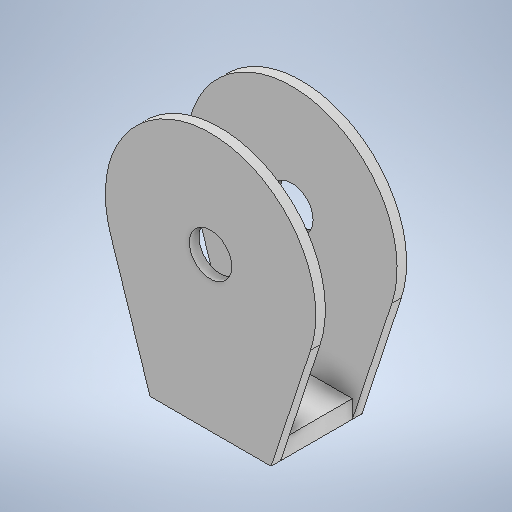
# Autodesk Inventor part: pulley
Saved by Autodesk Inventor 2025.2 (Build 292293000, 293)
## iProperties
Created: 2024-11-20
Part Number: pulley
Material: Generic
Document SubType Name: Modeling
Designer: email
Density: 1 g/cm^3
Appearance: Default
Author: email
Autodesk Inventor part; units mm, degrees
ref_plane "YZ Plane" through (0, 0, 0) normal (1, 0, 0) x (0, 1, 0)
ref_plane "XZ Plane" through (0, 0, 0) normal (0, 1, 0) x (-1, 0, 0)
ref_plane "XY Plane" through (0, 0, 0) normal (0, 0, 1) x (1, 0, 0)
sketch "Sketch1" plane through (0, 0, 0) normal (0, 0, 1) x (1, 0, 0)
  line L0 (0, 0) -> (25.3, 0)
  line L1 (25.3, 0) -> (25.3, 16.2986) construction
  line L2 (25.3, 16.2986) -> (0, 16.2986) construction
  line L3 (0, 16.2986) -> (0, 0) construction
  circle A0 centre (12.65, 32) radius 4.45
  circle A1 centre (12.65, 32) radius 22
  line L4 (25.3, 0) -> (33.5525, 25.138)
  line L5 (0, 0) -> (-8.2525, 25.138)
  line L6 (12.65, 54) -> (12.65, 0)
  dimension "d0" = 25.3
  dimension "d1" = 8.9
  dimension "d2" = 32
  dimension "d3" = 44
  dimension "d16" = 12.65
  constraints: 14 end point, 3 point on circle, 2 centre point, 2 parallel, 2 perpendicular, 2 tangent, 1 coincident, 1 horizontal, 1 midpoint, 1 point on line
  measures "d0" distance between parallel lines of L1 L3
  measures "d1" diameter of A0
  measures "d2" distance from line of L0 A0.centre
  measures "d3" diameter of A1
  measures "d16" distance between parallel lines of L1 L6
extrude "Extrusion1" add sketch "Sketch1" along normal blind 2 contours L5 A1 L6 L0 | L6 A1 L4 L0 | A1 L6 A0 | L6 A0 A1
sketch "Sketch2" plane through (0, 0, 2) normal (0, 0, 1) x (1, 0, 0)
  line L0 (-8.2525, 25.138) -> (0, 0) projected
  line L1 (0, 0) -> (25.3, 0)
  line L2 (25.3, 0) -> (25.3, 3.75)
  line L3 (25.3, 3.75) -> (0, 3.75)
  line L4 (0, 3.75) -> (0, 0)
  dimension "d6" = 25.3
  dimension "d7" = 3.75
  constraints: 8 end point, 2 parallel, 1 horizontal, 1 perpendicular
  measures "d6" distance between parallel lines of L2 L4
  measures "d7" distance of L1.end L2.end
extrude "Extrusion2" add sketch "Sketch2" along normal blind 7.5
mirror "Mirror1" about plane through (12.65, 1.875, 9.5) normal (0, 0, 1) of "Extrusion1", "Extrusion2"
sketch "Sketch3" plane through (0, 0, 0) normal (0, -1, 0) x (1, 0, 0)
  line L0 (0, 0) -> (12.65, 0)
  line L1 (12.65, 0) -> (12.65, 9.5)
  line L2 (12.65, 9.5) -> (0, 9.5)
  line L3 (0, 9.5) -> (0, 0)
  circle A0 centre (12.65, 9.5) radius 5
  dimension "d10" = 9.5
  dimension "d11" = 12.65
  dimension "d12" = 10
  constraints: 8 end point, 2 parallel, 1 centre point, 1 coincident, 1 horizontal, 1 perpendicular
  measures "d10" distance of L0.end L1.end
  measures "d11" distance of L1.end L2.end
  measures "d12" diameter of A0
extrude "Extrusion3" cut sketch "Sketch3" against normal blind 7.5 contours A0 L2 L1 | L1 L2 A0
body "Solid1"
